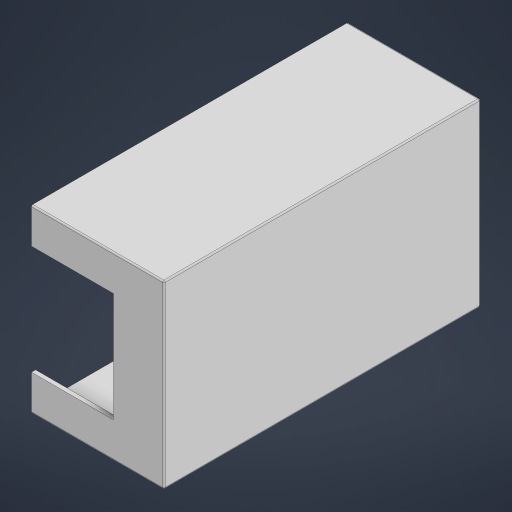
# Autodesk Inventor part: carcasa_exterior
Saved by Autodesk Inventor 2023.1 (Build 271208000, 208)
## iProperties
Created: 2022-12-06
Part Number: carcasa_exterior
Material: Generic
Document SubType Name: Modeling
Designer: amtat
Density: 1 g/cm^3
Appearance: Default
Author: amtat
Autodesk Inventor part; units mm, degrees
ref_plane "YZ Plane" through (0, 0, 0) normal (1, 0, 0) x (0, 1, 0)
ref_plane "XZ Plane" through (0, 0, 0) normal (0, 1, 0) x (-1, 0, 0)
ref_plane "XY Plane" through (0, 0, 0) normal (0, 0, 1) x (1, 0, 0)
sketch "Sketch1" plane through (0, 0, 0) normal (1, 0, 0) x (0, 1, 0)
  line L0 (0, 0) -> (63, 0)
  line L1 (63, 0) -> (63, -113)
  line L2 (63, -113) -> (0, -113)
  line L3 (0, -113) -> (0, 0)
  line L4 (0, 0) -> (-1.5, 0)
  line L5 (-1.5, 0) -> (-1.5, 1.5)
  line L6 (-1.5, 1.5) -> (64.5, 1.5)
  line L7 (64.5, 1.5) -> (64.5, -114.5)
  line L8 (64.5, -114.5) -> (-1.5, -114.5)
  line L9 (-1.5, -114.5) -> (-1.5, 1.5)
  dimension "d0" = 63
  dimension "d1" = 113
  dimension "d2" = 1.5
  dimension "d3" = 1.5
  dimension "d4" = 66
  dimension "d5" = 116
  constraints: 20 end point, 4 parallel, 3 horizontal, 3 perpendicular
  measures "d0" distance of L1.end L2.end
  measures "d1" distance of L0.end L1.end
  measures "d2" distance of L0.start L4.end
  measures "d3" distance of L4.end L5.end
  measures "d4" distance of L7.end L8.end
  measures "d5" distance of L6.end L7.end
extrude "Extrusion1" add sketch "Sketch1" along normal blind 47
sketch "Sketch2" plane through (47, 0, 0) normal (1, 0, 0) x (0, 0, -1)
  line L0 (114.5, -1.5) -> (114.5, 64.5) projected
  line L1 (114.5, 64.5) -> (-1.5, 64.5) projected
  line L2 (-1.5, 64.5) -> (-1.5, -1.5) projected
  line L3 (-1.5, -1.5) -> (114.5, -1.5) projected
  line L4 (0, 0) -> (0, 63) projected
  line L5 (0, 63) -> (113, 63) projected
  line L6 (113, 63) -> (113, 0) projected
  line L7 (113, 0) -> (0, 0) projected
extrude "Extrusion2" add sketch "Sketch2" along normal blind 1.5 contours L3 L2 L1 L0 | L4 L5 L6 L7
sketch "Sketch3" plane through (0, -1.5, 1.5) normal (0, 0, 1) x (1, 0, 0)
  line L0 (0, 66) -> (0, 0) projected
  line L1 (0, 0) -> (48.5, 0) projected
  line L2 (48.5, 66) -> (48.5, 0) projected
  line L3 (0, 66) -> (48.5, 66) projected
  line L4 (0, 0) -> (0, 66) projected
  line L5 (0, 66) -> (0, 33)
  line L6 (0, 33) -> (0, 13)
  line L7 (0, 13) -> (30, 13)
  line L8 (30, 13) -> (30, 53)
  line L9 (30, 53) -> (0, 53)
  point P0 (0, 1.5)
  dimension "d10" = 33
  dimension "d11" = 20
  dimension "d12" = 30
  dimension "d13" = 90
  dimension "d14" = 40
  constraints: 10 end point, 3 perpendicular, 2 point on line, 1 midpoint
  measures "d10" distance of L0.start L5.end
  measures "d11" distance of L5.end L6.end
  measures "d12" distance of L6.end L7.end
  measures "d13" angle of L7 L6
  measures "d14" distance of L7.end L8.end
extrude "Extrusion3" cut sketch "Sketch3" against normal blind 1.5 contours L9 L8 L7 L0
sketch "Sketch4" plane through (0, -1.5, -114.5) normal (0, 0, -1) x (-1, 0, 0)
  line L0 (0, 0) -> (0, 66) projected
  line L1 (0, 66) -> (-48.5, 66) projected
  line L2 (-48.5, 0) -> (-48.5, 66) projected
  line L3 (0, 0) -> (-48.5, 0) projected
  line L4 (0, 0) -> (-48.5, 0) projected
  line L5 (0, 0) -> (0, 33)
  line L6 (0, 33) -> (0, 40.5)
  line L7 (0, 40.5) -> (-20, 40.5)
  line L8 (-20, 40.5) -> (-20, 25.5)
  line L9 (-20, 25.5) -> (0, 25.5)
  line L10 (0, 64.5) -> (0, 1.5) projected
  line L11 (0, 33) -> (0, 25.5)
  dimension "d17" = 33
  dimension "d18" = 7.5
  dimension "d19" = 20
  dimension "d20" = 15
  constraints: 12 end point, 3 perpendicular, 2 point on line, 1 collinear, 1 midpoint
  measures "d17" distance of L0.start L5.end
  measures "d18" distance of L5.end L6.end
  measures "d19" distance of L6.end L7.end
  measures "d20" distance of L7.end L8.end
extrude "Extrusion4" cut sketch "Sketch4" against normal blind 1.5 contours L9 L8 L7 L0
fillet "Fillet1" radius 0.5 8 edges at (24.25, -1.5, -114.5) (48.5, 31.5, -114.5) (48.5, -1.5, -56.5) (48.5, 31.5, 1.5) (24.25, -1.5, 1.5) (24.25, 64.5, -114.5) (48.5, 64.5, -56.5) (24.25, 64.5, 1.5)
body "Solid1"
